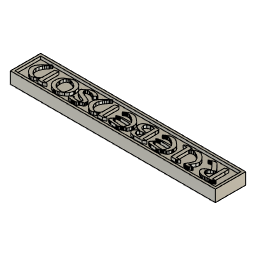
RuebensonBrandingIron v5 (Autodesk Fusion 360 design; units mm, degrees)
Autodesk Fusion 360 part; units mm, degrees
(part 1 of 2)
sketch "Sketch1" plane through (0, 0, 0) normal (0, 0, 1) x (1, 0, 0)
  line L0 (0, 0) -> (223.52, 0)
  line L1 (223.52, 0) -> (223.52, 33.02)
  line L2 (223.52, 33.02) -> (0, 33.02)
  line L3 (0, 33.02) -> (0, 0)
  dimension "d1" = 223.52
  dimension "d2" = 33.02
  constraint horizontal L0
  constraint vertical L1
  constraint horizontal L2
  constraint vertical L3
  constraint coincident L0.start L3.end
  measures "d1" distance of L0.start L0.end
  measures "d2" distance of L0.start L2.end
extrude "Extrude1" add sketch "Sketch1" along normal blind 12.7
sketch "Sketch4" plane through (0, 0, 12.7) normal (0, 0, 1) x (-1, 0, 0)
  line L0 (0, -33.02) -> (0, 0)
  line L1 (0, 0) -> (-223.52, 0)
  line L2 (-223.52, 0) -> (-223.52, -33.02)
  line L3 (-223.52, -33.02) -> (0, -33.02)
  spline S0 degree 3 poles (-115.0505, -8.6824) (-114.8396, -8.6121) (-114.6287, -8.533) (-114.4177, -8.4451) knots 0 0 0 0 1 1 1 1
  spline S1 degree 3 poles (-110.8582, -6.4148) (-110.7879, -6.3973) (-110.7132, -6.3885) (-110.6341, -6.3885) knots 0 0 0 0 1 1 1 1
  spline S2 degree 3 poles (-114.4177, -8.4451) (-114.2068, -8.3572) (-114.0047, -8.2693) (-113.8113, -8.1814) knots 0 0 0 0 1 1 1 1
  line L4 (-132.9807, -8.1814) -> (-132.9807, -14.2985)
  spline S3 degree 3 poles (-109.6322, -6.4148) (-109.3597, -6.4324) (-109.0741, -6.4588) (-108.7753, -6.4939) knots 0 0 0 0 1 1 1 1
  spline S4 degree 3 poles (-131.3855, -15.8805) (-131.5525, -15.8629) (-131.7239, -15.8541) (-131.8997, -15.8541) knots 0 0 0 0 1 1 1 1
  spline S5 degree 3 poles (-130.0276, -14.3249) (-129.0784, -14.2546) (-128.1952, -14.0173) (-127.3778, -13.613) knots 0 0 0 0 1 1 1 1
  line L5 (-132.9807, -23.395) -> (-132.9807, -23.4082)
  spline S6 degree 3 poles (-130.7923, -14.3249) (-130.6692, -14.3424) (-130.5418, -14.3468) (-130.41, -14.3381) knots 0 0 0 0 1 1 1 1
  line L6 (-136.4084, -24.7661) -> (-136.4084, -24.7397)
  line L7 (-132.9807, -15.775) -> (-132.9807, -23.3159)
  spline S7 degree 3 poles (-116.6325, -9.2229) (-116.1404, -9.0735) (-115.613, -8.8933) (-115.0505, -8.6824) knots 0 0 0 0 1 1 1 1
  line L8 (-131.0032, -8.2078) -> (-132.9807, -8.1814)
  arc A0 (-108.7753, -6.4939) -> (-108.5643, -6.5335) centre (-108.3426, -4.7686) ccw
  line L9 (-132.9807, -23.3555) -> (-132.9807, -23.395)
  line L10 (-131.8997, -15.8278) -> (-132.9807, -15.775)
  spline S8 degree 3 poles (-133.719, -25.9262) (-134.967, -25.9438) (-135.7273, -25.9131) (-135.9997, -25.834) knots 0 0 0 0 1 1 1 1
  line L11 (-131.8997, -15.8541) -> (-131.8997, -15.8278)
  spline S9 degree 3 poles (-113.8113, -8.1814) (-113.6179, -8.0759) (-113.4246, -7.9617) (-113.2312, -7.8386) knots 0 0 0 0 1 1 1 1
  spline S10 degree 3 poles (-132.9807, -23.5664) (-132.9807, -23.6279) (-132.9719, -23.6851) (-132.9544, -23.7378) knots 0 0 0 0 1 1 1 1
  arc A1 (-131.3855, -15.8805) -> (-130.8714, -15.9332) centre (-120.9987, 82.8585) ccw
  spline S11 degree 3 poles (-113.2312, -7.8386) (-113.0379, -7.7156) (-112.8533, -7.5926) (-112.6775, -7.4695) knots 0 0 0 0 1 1 1 1
  line L12 (-125.9935, -11.5827) -> (-125.9935, -11.5168)
  spline S12 degree 3 poles (-110.3836, -6.3885) (-110.1551, -6.3885) (-109.9046, -6.3973) (-109.6322, -6.4148) knots 0 0 0 0 1 1 1 1
  spline S13 degree 3 poles (-125.9672, -11.3191) (-125.9672, -10.4226) (-126.3715, -9.7283) (-127.18, -9.2361) knots 0 0 0 0 1 1 1 1
  line L13 (-117.4499, -9.4998) -> (-117.5026, -9.5261)
  line L14 (-132.9807, -23.4082) -> (-132.9807, -23.4214)
  line L15 (-133.1653, -25.9262) -> (-133.4553, -25.9262)
  spline S14 degree 3 poles (-125.9935, -11.5168) (-125.9935, -11.4904) (-125.9847, -11.4685) (-125.9672, -11.4509) knots 0 0 0 0 1 1 1 1
  line L16 (-132.9807, -14.2985) -> (-130.7923, -14.3249)
  line L17 (-110.6341, -6.3885) -> (-110.3836, -6.3885)
  spline S15 degree 3 poles (-130.41, -14.3381) (-130.2781, -14.3293) (-130.1507, -14.3249) (-130.0276, -14.3249) knots 0 0 0 0 1 1 1 1
  spline S16 degree 3 poles (-127.3778, -13.613) (-126.5604, -13.2087) (-126.099, -12.5319) (-125.9935, -11.5827) knots 0 0 0 0 1 1 1 1
  spline S17 degree 3 poles (-117.5026, -9.5261) (-117.4148, -9.4734) (-117.1247, -9.3723) (-116.6325, -9.2229) knots 0 0 0 0 1 1 1 1
  line L18 (-132.9807, -23.4214) -> (-132.9807, -23.5664)
  line L19 (-132.9807, -23.3159) -> (-132.9807, -23.3555)
  spline S18 degree 3 poles (-111.6888, -6.7708) (-111.3812, -6.5511) (-111.1043, -6.4324) (-110.8582, -6.4148) knots 0 0 0 0 1 1 1 1
  spline S19 degree 3 poles (-112.6775, -7.4695) (-112.326, -7.2234) (-111.9964, -6.9905) (-111.6888, -6.7708) knots 0 0 0 0 1 1 1 1
  arc A2 (-132.9544, -23.7378) -> (-132.9016, -23.9355) centre (-126.9769, -22.2497) ccw
  line L20 (-124.2533, -20.9166) -> (-124.2533, -20.8243)
  spline S20 degree 3 poles (-123.6601, -23.54) (-125.62, -24.6387) (-127.7777, -25.3637) (-130.1331, -25.7153) knots 0 0 0 0 1 1 1 1
  line L21 (-131.7151, -24.3179) -> (-128.7884, -24.2915)
  spline S21 degree 3 poles (-124.2533, -20.7584) (-124.3588, -19.0885) (-125.0883, -17.902) (-126.4418, -17.1988) knots 0 0 0 0 1 1 1 1
  line L22 (-124.2533, -20.8243) -> (-124.2533, -20.7584)
  line L23 (-137.2785, -6.2303) -> (-128.4456, -6.0984)
  spline S22 degree 3 poles (-131.6624, -25.8735) (-132.1721, -25.9087) (-132.6731, -25.9262) (-133.1653, -25.9262) knots 0 0 0 0 1 1 1 1
  spline S23 degree 3 poles (-126.4418, -17.1988) (-127.7953, -16.4957) (-129.2718, -16.0739) (-130.8714, -15.9332) knots 0 0 0 0 1 1 1 1
  line L24 (-133.4553, -25.9262) -> (-133.719, -25.9262)
  spline S24 degree 3 poles (-125.5453, -23.2368) (-124.684, -22.604) (-124.2533, -21.8306) (-124.2533, -20.9166) knots 0 0 0 0 1 1 1 1
  line L25 (-131.847, -24.3179) -> (-131.781, -24.3179)
  spline S25 degree 3 poles (-128.7884, -24.2915) (-128.7181, -24.3091) (-128.6478, -24.3179) (-128.5775, -24.3179) knots 0 0 0 0 1 1 1 1
  spline S26 degree 3 poles (-132.9016, -23.9355) (-132.884, -23.9971) (-132.8577, -24.0454) (-132.8225, -24.0806) knots 0 0 0 0 1 1 1 1
  spline S27 degree 3 poles (-132.4138, -24.2915) (-132.2468, -24.3091) (-132.0667, -24.3179) (-131.8733, -24.3179) knots 0 0 0 0 1 1 1 1
  line L26 (-131.781, -24.3179) -> (-131.7151, -24.3179)
  spline S28 degree 3 poles (-132.8225, -24.0806) (-132.7171, -24.2036) (-132.5808, -24.2739) (-132.4138, -24.2915) knots 0 0 0 0 1 1 1 1
  spline S29 degree 3 poles (-128.3665, -24.2915) (-127.347, -24.2212) (-126.4066, -23.8696) (-125.5453, -23.2368) knots 0 0 0 0 1 1 1 1
  arc A3 (-131.6624, -25.8735) -> (-130.1331, -25.7153) centre (-133.2155, -3.3893) ccw
  spline S30 degree 3 poles (-135.9997, -25.834) (-136.2722, -25.7549) (-136.4084, -25.3989) (-136.4084, -24.7661) knots 0 0 0 0 1 1 1 1
  spline S31 degree 3 poles (-127.9579, -6.138) (-127.7909, -6.1468) (-127.6283, -6.16) (-127.4701, -6.1775) knots 0 0 0 0 1 1 1 1
  spline S32 degree 3 poles (-128.5775, -24.3179) (-128.5072, -24.3179) (-128.4369, -24.3091) (-128.3665, -24.2915) knots 0 0 0 0 1 1 1 1
  line L27 (-131.8733, -24.3179) -> (-131.847, -24.3179)
  spline S33 degree 3 poles (-127.4701, -6.1775) (-126.2748, -6.283) (-125.1674, -6.6346) (-124.1479, -7.2322) knots 0 0 0 0 1 1 1 1
  line L28 (-136.4348, -21.6021) -> (-136.5402, -8.1023)
  spline S34 degree 3 poles (-161.1168, -9.5657) (-161.0992, -9.5569) (-161.0817, -9.5437) (-161.0641, -9.5261) knots 0 0 0 0 1 1 1 1
  line L29 (-140.7325, -8.1814) -> (-137.2785, -6.2303)
  arc A4 (-115.5251, -12.6901) -> (-115.6042, -13.3229) centre (-107.8557, -13.9702) ccw
  spline S35 degree 3 poles (-114.9055, -10.1853) (-115.1956, -10.9587) (-115.4021, -11.7937) (-115.5251, -12.6901) knots 0 0 0 0 1 1 1 1
  spline S36 degree 3 poles (-109.2103, -22.1953) (-108.8324, -22.4151) (-108.4501, -22.6128) (-108.0633, -22.7886) knots 0 0 0 0 1 1 1 1
  spline S37 degree 3 poles (-110.3836, -21.4966) (-109.9793, -21.7427) (-109.5882, -21.9756) (-109.2103, -22.1953) knots 0 0 0 0 1 1 1 1
  spline S38 degree 3 poles (-115.6042, -13.3229) (-115.6218, -13.5339) (-115.6306, -13.736) (-115.6306, -13.9294) knots 0 0 0 0 1 1 1 1
  spline S39 degree 3 poles (-112.8357, -19.5455) (-112.4666, -19.897) (-112.0755, -20.2398) (-111.6624, -20.5738) knots 0 0 0 0 1 1 1 1
  spline S40 degree 3 poles (-111.6624, -20.5738) (-111.2493, -20.9078) (-110.8231, -21.2154) (-110.3836, -21.4966) knots 0 0 0 0 1 1 1 1
  spline S41 degree 3 poles (-114.8923, -17.1197) (-114.699, -17.4361) (-114.4221, -17.8053) (-114.0618, -18.2271) knots 0 0 0 0 1 1 1 1
  line L30 (-136.4084, -24.7397) -> (-136.4348, -21.6021)
  line L31 (-161.0641, -9.5261) -> (-161.0641, -9.4998)
  line L32 (-136.5402, -8.1023) -> (-140.7325, -8.1814)
  spline S42 degree 3 poles (-161.1696, -9.6052) (-161.152, -9.5876) (-161.1344, -9.5745) (-161.1168, -9.5657) knots 0 0 0 0 1 1 1 1
  arc A5 (-162.7252, -14.7467) -> (-162.7516, -15.1686) centre (-159.3535, -15.1692) ccw
  spline S43 degree 3 poles (-113.9168, -8.7878) (-114.2859, -8.946) (-114.6155, -9.4119) (-114.9055, -10.1853) knots 0 0 0 0 1 1 1 1
  spline S44 degree 3 poles (-162.6593, -14.0876) (-162.6329, -13.8591) (-162.5934, -13.6393) (-162.5406, -13.4284) knots 0 0 0 0 1 1 1 1
  spline S45 degree 3 poles (-162.5406, -13.4284) (-162.4, -12.6022) (-162.2023, -11.8288) (-161.9474, -11.1081) knots 0 0 0 0 1 1 1 1
  spline S46 degree 3 poles (-128.4456, -6.0984) (-128.2874, -6.116) (-128.1248, -6.1292) (-127.9579, -6.138) knots 0 0 0 0 1 1 1 1
  spline S47 degree 3 poles (-161.9474, -11.1081) (-161.6925, -10.3874) (-161.4332, -9.8865) (-161.1696, -9.6052) knots 0 0 0 0 1 1 1 1
  spline S48 degree 3 poles (-162.7252, -14.7467) (-162.7076, -14.5358) (-162.6856, -14.3161) (-162.6593, -14.0876) knots 0 0 0 0 1 1 1 1
  line L33 (-198.044, -26.0053) -> (-198.1231, -26.0053)
  spline S49 degree 3 poles (-9.0744, -10.9763) (-8.0549, -12.3649) (-7.5452, -13.8327) (-7.5452, -15.3795) knots 0 0 0 0 1 1 1 1
  spline S50 degree 3 poles (-203.1987, -21.9976) (-203.4184, -21.7691) (-203.6601, -21.5142) (-203.9237, -21.233) knots 0 0 0 0 1 1 1 1
  spline S51 degree 3 poles (-201.9199, -23.3159) (-202.1308, -23.105) (-202.3329, -22.8941) (-202.5263, -22.6831) knots 0 0 0 0 1 1 1 1
  spline S52 degree 3 poles (-202.4077, -16.9484) (-202.2055, -17.2032) (-202.0078, -17.4449) (-201.8144, -17.6734) knots 0 0 0 0 1 1 1 1
  spline S53 degree 3 poles (-8.2571, -18.3985) (-8.7317, -19.3741) (-9.259, -20.2486) (-9.8391, -21.022) knots 0 0 0 0 1 1 1 1
  spline S54 degree 3 poles (-202.5527, -22.6568) (-202.7636, -22.4458) (-202.9789, -22.2261) (-203.1987, -21.9976) knots 0 0 0 0 1 1 1 1
  spline S55 degree 3 poles (-204.1083, -5.8875) (-203.7216, -5.8875) (-203.2514, -5.9315) (-202.6977, -6.0193) knots 0 0 0 0 1 1 1 1
  spline S56 degree 3 poles (-22.0469, -9.1834) (-22.6797, -9.8162) (-23.1103, -10.5017) (-23.3388, -11.24) knots 0 0 0 0 1 1 1 1
  spline S57 degree 3 poles (-14.4928, -6.4017) (-13.8336, -6.6917) (-13.1525, -7.0828) (-12.4494, -7.575) knots 0 0 0 0 1 1 1 1
  line L34 (-194.8008, -24.0015) -> (-194.7481, -24.0015)
  spline S58 degree 3 poles (-196.9893, -10.449) (-196.9717, -10.5193) (-196.9629, -10.5896) (-196.9629, -10.6599) knots 0 0 0 0 1 1 1 1
  line L35 (-223.52, 0) -> (-223.52, -33.02)
  spline S59 degree 3 poles (-202.6977, -6.0193) (-202.144, -6.1072) (-201.5771, -6.2479) (-200.997, -6.4412) knots 0 0 0 0 1 1 1 1
  spline S60 degree 3 poles (-200.997, -6.4412) (-200.0654, -6.74) (-199.1997, -7.2102) (-198.3999, -7.8518) knots 0 0 0 0 1 1 1 1
  spline S61 degree 3 poles (-200.9707, -24.3706) (-201.0234, -24.3003) (-201.0717, -24.2388) (-201.1157, -24.186) knots 0 0 0 0 1 1 1 1
  line L36 (-194.9063, -24.0015) -> (-194.8536, -24.0015)
  spline S62 degree 3 poles (-205.453, -19.4664) (-205.4706, -19.4488) (-205.4926, -19.4224) (-205.5189, -19.3873) knots 0 0 0 0 1 1 1 1
  spline S63 degree 3 poles (-198.4263, -13.5866) (-199.4018, -14.2897) (-200.4697, -14.9137) (-201.6298, -15.4586) knots 0 0 0 0 1 1 1 1
  line L37 (-202.5263, -22.6831) -> (-202.5395, -22.6831)
  spline S64 degree 3 poles (-203.0536, -16.0914) (-202.8251, -16.4078) (-202.6098, -16.6935) (-202.4077, -16.9484) knots 0 0 0 0 1 1 1 1
  arc A6 (-201.6694, -17.8448) -> (-201.5244, -18.0162) centre (-200.5632, -17.0559) ccw
  arc A7 (-202.1176, -15.6959) -> (-202.6054, -15.9069) centre (-191.6517, -40.5679) ccw
  spline S65 degree 3 poles (-16.1935, -5.9666) (-15.7189, -5.9666) (-15.152, -6.1116) (-14.4928, -6.4017) knots 0 0 0 0 1 1 1 1
  arc A8 (-205.453, -19.4664) -> (-204.517, -20.5474) centre (191.9498, 323.6805) ccw
  spline S66 degree 3 poles (-193.7594, -23.8564) (-193.5045, -23.7773) (-193.2716, -23.6939) (-193.0606, -23.606) knots 0 0 0 0 1 1 1 1
  line L38 (-202.6054, -15.9069) -> (-203.0536, -16.0914)
  line L39 (-223.52, -33.02) -> (0, -33.02)
  arc A9 (-202.1176, -15.6959) -> (-201.6298, -15.4586) centre (-204.0555, -11.0925) ccw
  spline S67 degree 3 poles (-196.9629, -10.8708) (-196.9629, -11.9782) (-197.4507, -12.8835) (-198.4263, -13.5866) knots 0 0 0 0 1 1 1 1
  spline S68 degree 3 poles (-198.3999, -7.8518) (-197.6001, -8.4934) (-197.1299, -9.3591) (-196.9893, -10.449) knots 0 0 0 0 1 1 1 1
  spline S69 degree 3 poles (-194.5372, -24.0015) (-194.2735, -23.9839) (-194.0142, -23.9355) (-193.7594, -23.8564) knots 0 0 0 0 1 1 1 1
  arc A10 (-19.753, -7.9573) -> (-20.0166, -7.9968) centre (-19.4806, -10.6714) ccw
  line L40 (0, -33.02) -> (0, 0)
  spline S70 degree 3 poles (-20.0166, -7.9968) (-20.7373, -8.155) (-21.4141, -8.5505) (-22.0469, -9.1834) knots 0 0 0 0 1 1 1 1
  arc A11 (-19.4893, -7.9441) -> (-19.753, -7.9573) centre (-19.4891, -10.5923) ccw
  line L41 (-194.6426, -24.0015) -> (-194.5372, -24.0015)
  spline S71 degree 3 poles (-202.5395, -22.6831) (-202.5483, -22.6831) (-202.5527, -22.6743) (-202.5527, -22.6568) knots 0 0 0 0 1 1 1 1
  spline S72 degree 3 poles (-201.2607, -24.0278) (-201.4892, -23.7642) (-201.7089, -23.5269) (-201.9199, -23.3159) knots 0 0 0 0 1 1 1 1
  spline S73 degree 3 poles (-7.5452, -15.3795) (-7.5452, -16.4166) (-7.7825, -17.423) (-8.2571, -18.3985) knots 0 0 0 0 1 1 1 1
  line L42 (-197.9649, -26.0053) -> (-198.044, -26.0053)
  line L43 (-197.8989, -26.0053) -> (-197.9649, -26.0053)
  line L44 (-196.9629, -10.6599) -> (-196.9629, -10.8708)
  spline S74 degree 3 poles (-9.8391, -21.022) (-10.2258, -21.5318) (-10.5949, -21.9756) (-10.9465, -22.3535) knots 0 0 0 0 1 1 1 1
  line L45 (0, 0) -> (-223.52, 0)
  spline S75 degree 3 poles (-12.4494, -7.575) (-11.2189, -8.4539) (-10.0939, -9.5876) (-9.0744, -10.9763) knots 0 0 0 0 1 1 1 1
  arc A12 (-201.6694, -17.8448) -> (-201.8144, -17.6734) centre (-202.7756, -18.6338) ccw
  spline S76 degree 3 poles (-199.7182, -25.4516) (-200.1841, -25.1177) (-200.6015, -24.7573) (-200.9707, -24.3706) knots 0 0 0 0 1 1 1 1
  spline S77 degree 3 poles (-198.1231, -26.0053) (-198.7207, -25.9702) (-199.2524, -25.7856) (-199.7182, -25.4516) knots 0 0 0 0 1 1 1 1
  spline S78 degree 3 poles (-201.1157, -24.186) (-201.1596, -24.1333) (-201.208, -24.0806) (-201.2607, -24.0278) knots 0 0 0 0 1 1 1 1
  line L46 (-194.7481, -24.0015) -> (-194.6426, -24.0015)
  spline S79 degree 3 poles (-203.9237, -21.233) (-204.0292, -21.1099) (-204.227, -20.8814) (-204.517, -20.5474) knots 0 0 0 0 1 1 1 1
  line L47 (-194.959, -24.0015) -> (-194.9063, -24.0015)
  spline S80 degree 3 poles (-195.9082, -23.7642) (-195.6446, -23.9048) (-195.3282, -23.9839) (-194.959, -24.0015) knots 0 0 0 0 1 1 1 1
  line L48 (-194.8536, -24.0015) -> (-194.8008, -24.0015)
  spline S81 degree 3 poles (-23.3388, -11.24) (-23.374, -11.3982) (-23.4048, -11.552) (-23.4311, -11.7014) knots 0 0 0 0 1 1 1 1
  line L49 (-204.1479, -5.8875) -> (-204.1083, -5.8875)
  spline S82 degree 3 poles (-196.9102, -22.9204) (-196.875, -22.9907) (-196.8355, -23.0435) (-196.7915, -23.0786) knots 0 0 0 0 1 1 1 1
  spline S83 degree 3 poles (-196.7915, -23.0786) (-196.7476, -23.1138) (-196.708, -23.1577) (-196.6729, -23.2105) knots 0 0 0 0 1 1 1 1
  arc A13 (-199.4414, -20.3497) -> (-198.8086, -20.9957) centre (-167.4667, 10.3396) ccw
  spline S84 degree 3 poles (-67.3132, -8.3923) (-67.1902, -8.3045) (-67.0628, -8.2078) (-66.9309, -8.1023) knots 0 0 0 0 1 1 1 1
  spline S85 degree 3 poles (-196.6729, -23.2105) (-196.4268, -23.439) (-196.1719, -23.6235) (-195.9082, -23.7642) knots 0 0 0 0 1 1 1 1
  spline S86 degree 3 poles (-70.4772, -10.1062) (-70.4245, -10.071) (-70.363, -10.0271) (-70.2927, -9.9744) knots 0 0 0 0 1 1 1 1
  spline S87 degree 3 poles (-200.8652, -18.7677) (-200.6367, -19.0225) (-200.3906, -19.2994) (-200.1269, -19.5982) knots 0 0 0 0 1 1 1 1
  arc A14 (-66.9309, -8.1023) -> (-66.5486, -7.7859) centre (-76.0785, 3.3402) ccw
  line L50 (-88.8919, -12.1364) -> (-88.8919, -24.6079)
  spline S88 degree 3 poles (-68.6052, -15.4455) (-68.6228, -15.4367) (-68.6404, -15.4235) (-68.6579, -15.4059) knots 0 0 0 0 1 1 1 1
  spline S89 degree 3 poles (-68.6579, -15.4059) (-69.0974, -15.2301) (-69.5061, -15.028) (-69.884, -14.7995) knots 0 0 0 0 1 1 1 1
  spline S90 degree 3 poles (-59.2714, -20.8375) (-59.3417, -20.5738) (-59.4296, -20.3145) (-59.535, -20.0596) knots 0 0 0 0 1 1 1 1
  line L51 (-198.769, -21.0088) -> (-198.7559, -21.022)
  spline S91 degree 3 poles (-70.1081, -24.8716) (-70.4948, -24.6958) (-70.8156, -24.5156) (-71.0705, -24.3311) knots 0 0 0 0 1 1 1 1
  spline S92 degree 3 poles (-70.2927, -9.9744) (-70.0114, -9.8337) (-69.6071, -9.658) (-69.0798, -9.447) knots 0 0 0 0 1 1 1 1
  spline S93 degree 3 poles (-60.6424, -18.8336) (-60.9413, -18.6226) (-61.5916, -18.315) (-62.5936, -17.9107) knots 0 0 0 0 1 1 1 1
  spline S94 degree 3 poles (-65.6389, -26.1372) (-65.9466, -26.102) (-66.2498, -26.0581) (-66.5486, -26.0053) knots 0 0 0 0 1 1 1 1
  spline S95 degree 3 poles (-69.0007, -20.9693) (-68.9831, -20.9341) (-68.9612, -20.9034) (-68.9348, -20.877) knots 0 0 0 0 1 1 1 1
  spline S96 degree 3 poles (-68.5525, -15.4323) (-68.57, -15.4498) (-68.5876, -15.4542) (-68.6052, -15.4455) knots 0 0 0 0 1 1 1 1
  spline S97 degree 3 poles (-64.7293, -26.1899) (-65.0281, -26.1899) (-65.3313, -26.1723) (-65.6389, -26.1372) knots 0 0 0 0 1 1 1 1
  line L52 (-197.3584, -22.4722) -> (-196.9102, -22.9204)
  spline S98 degree 3 poles (-58.5067, -10.0271) (-58.5946, -9.8162) (-58.9154, -9.6316) (-59.4691, -9.4734) knots 0 0 0 0 1 1 1 1
  spline S99 degree 3 poles (-66.5486, -26.0053) (-67.2166, -25.8999) (-67.8581, -25.7417) (-68.4734, -25.5307) knots 0 0 0 0 1 1 1 1
  spline S100 degree 3 poles (-200.1269, -19.5982) (-199.8808, -19.8795) (-199.6523, -20.1299) (-199.4414, -20.3497) knots 0 0 0 0 1 1 1 1
  spline S101 degree 3 poles (-65.3885, -6.8499) (-65.0193, -6.5599) (-64.6766, -6.3709) (-64.3602, -6.283) knots 0 0 0 0 1 1 1 1
  spline S102 degree 3 poles (-70.8596, -13.2702) (-70.9035, -12.9714) (-70.9343, -12.6638) (-70.9518, -12.3474) knots 0 0 0 0 1 1 1 1
  spline S103 degree 3 poles (-64.1624, -6.2698) (-64.0306, -6.261) (-63.8504, -6.2479) (-63.6219, -6.2303) knots 0 0 0 0 1 1 1 1
  spline S104 degree 3 poles (-68.4734, -25.5307) (-69.0886, -25.3198) (-69.6335, -25.1001) (-70.1081, -24.8716) knots 0 0 0 0 1 1 1 1
  spline S105 degree 3 poles (-59.4691, -9.4734) (-60.0228, -9.3152) (-60.6337, -9.1746) (-61.3016, -9.0515) knots 0 0 0 0 1 1 1 1
  line L53 (-64.5975, -26.1899) -> (-64.6238, -26.1899)
  line L54 (-64.3865, -26.1899) -> (-64.5447, -26.1899)
  line L55 (-64.3602, -6.283) -> (-64.1624, -6.2698)
  spline S106 degree 3 poles (-68.8689, -20.8111) (-68.781, -20.7408) (-68.7019, -20.688) (-68.6316, -20.6529) knots 0 0 0 0 1 1 1 1
  spline S107 degree 3 poles (-66.5486, -7.7859) (-66.1443, -7.4519) (-65.7576, -7.1399) (-65.3885, -6.8499) knots 0 0 0 0 1 1 1 1
  spline S108 degree 3 poles (-68.6316, -20.6529) (-68.5613, -20.6177) (-68.4997, -20.6441) (-68.447, -20.732) knots 0 0 0 0 1 1 1 1
  spline S109 degree 3 poles (-58.4936, -10.0666) (-58.5023, -10.0578) (-58.5067, -10.0447) (-58.5067, -10.0271) knots 0 0 0 0 1 1 1 1
  spline S110 degree 3 poles (-59.535, -20.0596) (-59.6405, -19.8048) (-59.7811, -19.5894) (-59.9569, -19.4137) knots 0 0 0 0 1 1 1 1
  spline S111 degree 3 poles (-198.0967, -21.7076) (-197.8682, -21.9361) (-197.6221, -22.1909) (-197.3584, -22.4722) knots 0 0 0 0 1 1 1 1
  spline S112 degree 3 poles (-68.447, -20.732) (-68.4294, -20.7496) (-68.4206, -20.7715) (-68.4206, -20.7979) knots 0 0 0 0 1 1 1 1
  spline S113 degree 3 poles (-63.4901, -26.1504) (-63.7186, -26.1591) (-63.9647, -26.1723) (-64.2283, -26.1899) knots 0 0 0 0 1 1 1 1
  spline S114 degree 3 poles (-70.6618, -14.0348) (-70.7497, -13.8239) (-70.8156, -13.569) (-70.8596, -13.2702) knots 0 0 0 0 1 1 1 1
  spline S115 degree 3 poles (-71.0705, -24.3311) (-71.3254, -24.1465) (-71.4704, -23.9927) (-71.5055, -23.8696) knots 0 0 0 0 1 1 1 1
  spline S116 degree 3 poles (-59.1659, -21.4834) (-59.1835, -21.2813) (-59.2186, -21.066) (-59.2714, -20.8375) knots 0 0 0 0 1 1 1 1
  spline S117 degree 3 poles (-70.6091, -10.2117) (-70.5739, -10.1765) (-70.53, -10.1413) (-70.4772, -10.1062) knots 0 0 0 0 1 1 1 1
  spline S118 degree 3 poles (-198.7559, -21.022) (-198.5449, -21.2505) (-198.3252, -21.479) (-198.0967, -21.7076) knots 0 0 0 0 1 1 1 1
  line L56 (-88.8919, -24.6079) -> (-92.4251, -25.9262)
  spline S119 degree 3 poles (-59.9569, -19.4137) (-60.1151, -19.2379) (-60.3436, -19.0445) (-60.6424, -18.8336) knots 0 0 0 0 1 1 1 1
  line L57 (-71.5055, -23.8301) -> (-71.5055, -23.8169)
  spline S120 degree 3 poles (-69.884, -14.7995) (-70.2619, -14.571) (-70.5212, -14.3161) (-70.6618, -14.0348) knots 0 0 0 0 1 1 1 1
  line L58 (-64.6766, -26.1899) -> (-64.7293, -26.1899)
  spline S121 degree 3 poles (-88.8524, -11.7014) (-88.8788, -11.8508) (-88.8919, -11.9958) (-88.8919, -12.1364) knots 0 0 0 0 1 1 1 1
  spline S122 degree 3 poles (-59.1395, -22.0503) (-59.1395, -21.8745) (-59.1483, -21.6856) (-59.1659, -21.4834) knots 0 0 0 0 1 1 1 1
  line L59 (-70.7145, -10.2117) -> (-70.6091, -10.2117)
  spline S123 degree 3 poles (-198.8086, -20.9957) (-198.791, -20.9957) (-198.7778, -21.0001) (-198.769, -21.0088) knots 0 0 0 0 1 1 1 1
  spline S124 degree 3 poles (-69.0798, -9.447) (-68.5525, -9.2361) (-67.9636, -8.8845) (-67.3132, -8.3923) knots 0 0 0 0 1 1 1 1
  line L60 (-64.6238, -26.1899) -> (-64.6766, -26.1899)
  line L61 (-64.2283, -26.1899) -> (-64.3865, -26.1899)
  line L62 (-62.5936, -17.9107) -> (-68.5525, -15.4323)
  line L63 (-64.5447, -26.1899) -> (-64.5975, -26.1899)
  line L64 (-71.5055, -23.8696) -> (-71.5055, -23.8301)
  arc A15 (-63.4901, -26.1504) -> (-62.8045, -26.0844) centre (-63.7234, -20.1261) ccw
  line L65 (-68.9348, -20.877) -> (-68.8689, -20.8111)
  spline S125 degree 3 poles (-69.093, -21.0748) (-69.0666, -21.0396) (-69.0359, -21.0044) (-69.0007, -20.9693) knots 0 0 0 0 1 1 1 1
  spline S126 degree 3 poles (-69.1853, -21.1539) (-69.1501, -21.1363) (-69.1194, -21.1099) (-69.093, -21.0748) knots 0 0 0 0 1 1 1 1
  line L66 (-71.0441, -23.0654) -> (-70.9518, -22.9732)
  line L67 (-71.1364, -23.1577) -> (-71.0441, -23.0654)
  line L68 (-70.9518, -22.9732) -> (-69.1853, -21.1539)
  spline S127 degree 3 poles (-71.4396, -23.4741) (-71.3781, -23.3862) (-71.3034, -23.3071) (-71.2155, -23.2368) knots 0 0 0 0 1 1 1 1
  spline S128 degree 3 poles (-55.7382, -19.8619) (-55.7207, -19.897) (-55.7119, -19.9366) (-55.7119, -19.9805) knots 0 0 0 0 1 1 1 1
  spline S129 degree 3 poles (-56.8456, -17.1988) (-56.5644, -17.5504) (-56.3183, -17.9591) (-56.1074, -18.4249) knots 0 0 0 0 1 1 1 1
  spline S130 degree 3 poles (-58.744, -15.6432) (-57.9179, -16.1002) (-57.2851, -16.6188) (-56.8456, -17.1988) knots 0 0 0 0 1 1 1 1
  line L69 (-67.5769, -11.2927) -> (-67.5769, -11.3454)
  spline S131 degree 3 poles (-61.4334, -14.3776) (-60.4667, -14.7643) (-59.5702, -15.1862) (-58.744, -15.6432) knots 0 0 0 0 1 1 1 1
  line L70 (-65.4412, -12.8483) -> (-61.4334, -14.3776)
  spline S132 degree 3 poles (-67.0496, -12.0441) (-66.7507, -12.2639) (-66.2146, -12.5319) (-65.4412, -12.8483) knots 0 0 0 0 1 1 1 1
  spline S133 degree 3 poles (-71.176, -23.1841) (-71.1672, -23.1665) (-71.154, -23.1577) (-71.1364, -23.1577) knots 0 0 0 0 1 1 1 1
  line L71 (-71.5319, -23.7773) -> (-71.5319, -23.7642)
  spline S134 degree 3 poles (-71.5055, -23.8169) (-71.5231, -23.7993) (-71.5319, -23.7861) (-71.5319, -23.7773) knots 0 0 0 0 1 1 1 1
  spline S135 degree 3 poles (-56.1074, -18.4249) (-55.8964, -18.8907) (-55.7734, -19.3697) (-55.7382, -19.8619) knots 0 0 0 0 1 1 1 1
  spline S136 degree 3 poles (-71.2155, -23.2368) (-71.1979, -23.2193) (-71.1848, -23.2017) (-71.176, -23.1841) knots 0 0 0 0 1 1 1 1
  spline S137 degree 3 poles (-71.5319, -23.7642) (-71.5319, -23.6587) (-71.5012, -23.562) (-71.4396, -23.4741) knots 0 0 0 0 1 1 1 1
  line L72 (-55.7119, -19.9805) -> (-55.7119, -20.0992)
  spline S138 degree 3 poles (-58.5199, -10.3171) (-58.4936, -10.2644) (-58.4804, -10.2117) (-58.4804, -10.1589) knots 0 0 0 0 1 1 1 1
  spline S139 degree 3 poles (-67.5769, -11.4245) (-67.5242, -11.6179) (-67.3484, -11.8244) (-67.0496, -12.0441) knots 0 0 0 0 1 1 1 1
  line L73 (-67.5769, -11.2136) -> (-67.5769, -11.2927)
  line L74 (-67.5769, -11.0818) -> (-67.5769, -11.2136)
  spline S140 degree 3 poles (-60.7215, -25.0561) (-61.0731, -25.4077) (-61.3543, -25.6274) (-61.5653, -25.7153) knots 0 0 0 0 1 1 1 1
  line L75 (-67.6033, -10.7654) -> (-67.6033, -10.9367)
  arc A16 (-59.1264, -23.5269) -> (-59.5614, -23.9487) centre (-45.4173, -38.0996) ccw
  spline S141 degree 3 poles (-56.3974, -21.4571) (-56.749, -21.712) (-57.1445, -21.9888) (-57.5839, -22.2876) knots 0 0 0 0 1 1 1 1
  spline S142 degree 3 poles (-55.7514, -20.5342) (-55.7778, -20.6836) (-55.8085, -20.8287) (-55.8437, -20.9693) knots 0 0 0 0 1 1 1 1
  line L76 (-58.4804, -10.1589) -> (-58.4804, -10.1194)
  line L77 (-58.4804, -10.1194) -> (-58.4804, -10.0798)
  spline S143 degree 3 poles (-61.5653, -25.7153) (-61.7938, -25.8208) (-62.0091, -25.8999) (-62.2113, -25.9526) knots 0 0 0 0 1 1 1 1
  spline S144 degree 3 poles (-55.8437, -20.9693) (-55.8613, -21.0396) (-56.0458, -21.2022) (-56.3974, -21.4571) knots 0 0 0 0 1 1 1 1
  spline S145 degree 3 poles (-58.6781, -10.6467) (-58.6518, -10.5852) (-58.6298, -10.5281) (-58.6122, -10.4753) knots 0 0 0 0 1 1 1 1
  spline S146 degree 3 poles (-62.2113, -25.9526) (-62.4134, -26.0053) (-62.6112, -26.0493) (-62.8045, -26.0844) knots 0 0 0 0 1 1 1 1
  spline S147 degree 3 poles (-58.5858, -10.4753) (-58.5683, -10.4226) (-58.5463, -10.3699) (-58.5199, -10.3171) knots 0 0 0 0 1 1 1 1
  line L78 (-58.6122, -10.4753) -> (-58.5858, -10.4753)
  spline S148 degree 3 poles (-58.7177, -10.8181) (-58.7177, -10.7654) (-58.7045, -10.7082) (-58.6781, -10.6467) knots 0 0 0 0 1 1 1 1
  spline S149 degree 3 poles (-58.599, -23.0786) (-58.6254, -23.0962) (-58.6474, -23.1138) (-58.6649, -23.1314) knots 0 0 0 0 1 1 1 1
  spline S150 degree 3 poles (-58.1903, -22.7622) (-58.3134, -22.8501) (-58.4276, -22.938) (-58.5331, -23.0259) knots 0 0 0 0 1 1 1 1
  spline S151 degree 3 poles (-67.6033, -10.9367) (-67.6033, -10.9983) (-67.5945, -11.0466) (-67.5769, -11.0818) knots 0 0 0 0 1 1 1 1
  spline S152 degree 3 poles (-58.6649, -23.1314) (-58.8231, -23.2544) (-58.9769, -23.3862) (-59.1264, -23.5269) knots 0 0 0 0 1 1 1 1
  line L79 (-67.5769, -11.3454) -> (-67.5769, -11.4245)
  spline S153 degree 3 poles (-59.5614, -23.9487) (-59.9833, -24.3354) (-60.37, -24.7046) (-60.7215, -25.0561) knots 0 0 0 0 1 1 1 1
  spline S154 degree 3 poles (-57.8212, -22.4722) (-57.9442, -22.5777) (-58.0673, -22.6743) (-58.1903, -22.7622) knots 0 0 0 0 1 1 1 1
  spline S155 degree 3 poles (-57.7026, -22.3799) (-57.7465, -22.4063) (-57.786, -22.437) (-57.8212, -22.4722) knots 0 0 0 0 1 1 1 1
  spline S156 degree 3 poles (-67.5901, -10.4226) (-67.5989, -10.5456) (-67.6033, -10.6599) (-67.6033, -10.7654) knots 0 0 0 0 1 1 1 1
  spline S157 degree 3 poles (-58.5331, -23.0259) (-58.5507, -23.0435) (-58.5727, -23.0611) (-58.599, -23.0786) knots 0 0 0 0 1 1 1 1
  spline S158 degree 3 poles (-57.5839, -22.2876) (-57.6191, -22.3228) (-57.6586, -22.3535) (-57.7026, -22.3799) knots 0 0 0 0 1 1 1 1
  spline S159 degree 3 poles (-55.7119, -20.0992) (-55.7119, -20.2398) (-55.725, -20.3848) (-55.7514, -20.5342) knots 0 0 0 0 1 1 1 1
  line L80 (-58.4804, -10.0798) -> (-58.4936, -10.0666)
  spline S160 degree 3 poles (-57.2016, -9.7371) (-57.2631, -9.7898) (-57.3202, -9.8513) (-57.373, -9.9216) knots 0 0 0 0 1 1 1 1
  spline S161 degree 3 poles (-57.0038, -9.5789) (-57.0741, -9.6316) (-57.1401, -9.6843) (-57.2016, -9.7371) knots 0 0 0 0 1 1 1 1
  spline S162 degree 3 poles (-67.5242, -10.0535) (-67.5593, -10.1765) (-67.5813, -10.2995) (-67.5901, -10.4226) knots 0 0 0 0 1 1 1 1
  spline S163 degree 3 poles (-58.6254, -11.0027) (-58.6518, -10.9851) (-58.6737, -10.9499) (-58.6913, -10.8972) knots 0 0 0 0 1 1 1 1
  spline S164 degree 3 poles (-58.6913, -10.8576) (-58.6913, -10.8489) (-58.7001, -10.8357) (-58.7177, -10.8181) knots 0 0 0 0 1 1 1 1
  line L81 (-58.6913, -10.8972) -> (-58.6913, -10.8576)
  spline S165 degree 3 poles (-57.373, -9.9216) (-57.6542, -10.1853) (-57.8959, -10.4314) (-58.0981, -10.6599) knots 0 0 0 0 1 1 1 1
  spline S166 degree 3 poles (-58.0981, -10.6599) (-58.3002, -10.8884) (-58.454, -11.0114) (-58.5595, -11.029) knots 0 0 0 0 1 1 1 1
  spline S167 degree 3 poles (-58.5595, -11.029) (-58.5771, -11.029) (-58.599, -11.0202) (-58.6254, -11.0027) knots 0 0 0 0 1 1 1 1
  arc A17 (-212.8884, -6.4676) -> (-213.2444, -6.6258) centre (-207.3135, -19.4907) ccw
  spline S168 degree 3 poles (-214.365, -7.2058) (-214.2244, -7.118) (-214.0881, -7.0389) (-213.9563, -6.9685) knots 0 0 0 0 1 1 1 1
  spline S169 degree 3 poles (-214.6682, -7.3772) (-214.5715, -7.3157) (-214.4704, -7.2586) (-214.365, -7.2058) knots 0 0 0 0 1 1 1 1
  spline S170 degree 3 poles (-214.945, -7.5486) (-214.8572, -7.4959) (-214.7649, -7.4388) (-214.6682, -7.3772) knots 0 0 0 0 1 1 1 1
  arc A18 (-215.6174, -8.0364) -> (-215.9733, -8.2869) centre (-198.739, -32.3997) ccw
  spline S171 degree 3 poles (-212.8884, -6.4676) (-212.8357, -6.45) (-212.7786, -6.428) (-212.7171, -6.4017) knots 0 0 0 0 1 1 1 1
  spline S172 degree 3 poles (-201.5244, -18.0162) (-201.3134, -18.2623) (-201.0937, -18.5128) (-200.8652, -18.7677) knots 0 0 0 0 1 1 1 1
  arc A19 (-213.2444, -6.6258) -> (-213.574, -6.784) centre (-208.3418, -17.2619) ccw
  spline S173 degree 3 poles (-213.9563, -6.9685) (-213.8245, -6.8982) (-213.697, -6.8367) (-213.574, -6.784) knots 0 0 0 0 1 1 1 1
  line L82 (-212.0974, -26.0053) -> (-212.1502, -21.7603)
  spline S174 degree 3 poles (-215.2878, -7.7859) (-215.2351, -7.7508) (-215.178, -7.7156) (-215.1164, -7.6804) knots 0 0 0 0 1 1 1 1
  line L83 (-208.6434, -24.8188) -> (-212.0974, -26.0053)
  line L84 (-212.2293, -8.2605) -> (-215.9733, -8.2869)
  line L85 (-204.161, -5.8875) -> (-204.1479, -5.8875)
  spline S175 degree 3 poles (-215.1164, -7.6804) (-215.0549, -7.6453) (-214.9978, -7.6013) (-214.945, -7.5486) knots 0 0 0 0 1 1 1 1
  spline S176 degree 3 poles (-208.4325, -6.2435) (-207.9754, -6.1995) (-207.5272, -6.1512) (-207.0878, -6.0984) knots 0 0 0 0 1 1 1 1
  spline S177 degree 3 poles (-11.3683, -16.3024) (-11.3683, -15.1422) (-11.6672, -14.0568) (-12.2648, -13.0461) knots 0 0 0 0 1 1 1 1
  spline S178 degree 3 poles (-13.9523, -23.395) (-13.6359, -22.938) (-13.3546, -22.481) (-13.1085, -22.024) knots 0 0 0 0 1 1 1 1
  spline S179 degree 3 poles (-209.9617, -6.3357) (-209.3992, -6.3182) (-208.8895, -6.2874) (-208.4325, -6.2435) knots 0 0 0 0 1 1 1 1
  line L86 (-204.2006, -5.8875) -> (-204.161, -5.8875)
  spline S180 degree 3 poles (-210.6604, -6.3621) (-210.4407, -6.3621) (-210.2078, -6.3533) (-209.9617, -6.3357) knots 0 0 0 0 1 1 1 1
  line L87 (-19.3179, -7.9441) -> (-19.4893, -7.9441)
  spline S181 degree 3 poles (-211.8865, -6.3357) (-211.8338, -6.3533) (-211.7766, -6.3621) (-211.7151, -6.3621) knots 0 0 0 0 1 1 1 1
  line L88 (-212.5457, -6.3357) -> (-212.2029, -6.3357)
  spline S182 degree 3 poles (-18.0655, -8.2078) (-18.2061, -8.155) (-18.3687, -8.1067) (-18.5533, -8.0628) knots 0 0 0 0 1 1 1 1
  spline S183 degree 3 poles (-17.4063, -8.4187) (-17.4415, -8.4187) (-17.5162, -8.3967) (-17.6304, -8.3528) knots 0 0 0 0 1 1 1 1
  line L89 (-11.3683, -16.3683) -> (-11.3683, -16.3024)
  line L90 (-23.4707, -12.1364) -> (-23.4707, -24.6079)
  line L91 (-208.6434, -11.3191) -> (-208.6434, -24.8188)
  line L92 (-212.2029, -6.3357) -> (-211.8865, -6.3357)
  arc A20 (-215.6174, -8.0364) -> (-215.2878, -7.7859) centre (-218.2577, -4.2202) ccw
  spline S184 degree 3 poles (-19.1202, -7.9705) (-19.1905, -7.9529) (-19.2564, -7.9441) (-19.3179, -7.9441) knots 0 0 0 0 1 1 1 1
  line L93 (-211.5437, -6.3621) -> (-211.4251, -6.3621)
  line L94 (-211.3064, -6.3621) -> (-210.6604, -6.3621)
  line L95 (-211.7151, -6.3621) -> (-211.5437, -6.3621)
  line L96 (-208.617, -8.3396) -> (-208.6434, -11.3191)
  spline S185 degree 3 poles (-18.5533, -8.0628) (-18.7378, -8.0188) (-18.9268, -7.9881) (-19.1202, -7.9705) knots 0 0 0 0 1 1 1 1
  line L97 (-212.1502, -21.7603) -> (-212.2293, -8.2605)
  spline S186 degree 3 poles (-205.7562, -5.9798) (-205.2904, -5.9358) (-204.7851, -5.9051) (-204.2401, -5.8875) knots 0 0 0 0 1 1 1 1
  spline S187 degree 3 poles (-12.2648, -13.0461) (-12.8625, -12.0354) (-13.5128, -11.1872) (-14.2159, -10.5017) knots 0 0 0 0 1 1 1 1
  spline S188 degree 3 poles (-13.1085, -22.024) (-12.5812, -21.1275) (-12.1681, -20.2178) (-11.8693, -19.295) knots 0 0 0 0 1 1 1 1
  line L98 (-211.4251, -6.3621) -> (-211.3064, -6.3621)
  spline S189 degree 3 poles (-212.7171, -6.4017) (-212.6555, -6.3753) (-212.5984, -6.3533) (-212.5457, -6.3357) knots 0 0 0 0 1 1 1 1
  line L99 (-11.3683, -16.4606) -> (-11.3683, -16.3683)
  spline S190 degree 3 poles (-23.4311, -11.7014) (-23.4575, -11.8508) (-23.4707, -11.9958) (-23.4707, -12.1364) knots 0 0 0 0 1 1 1 1
  line L100 (-204.2401, -5.8875) -> (-204.2006, -5.8875)
  line L101 (-15.7452, -9.3679) -> (-17.4063, -8.4187)
  spline S191 degree 3 poles (-15.0069, -9.8425) (-15.2706, -9.6492) (-15.5167, -9.491) (-15.7452, -9.3679) knots 0 0 0 0 1 1 1 1
  spline S192 degree 3 poles (-11.8693, -19.295) (-11.5705, -18.3722) (-11.4035, -17.4274) (-11.3683, -16.4606) knots 0 0 0 0 1 1 1 1
  line L102 (-23.4707, -24.6079) -> (-27.0038, -25.9262)
  spline S193 degree 3 poles (-207.0878, -6.0984) (-206.6659, -6.0633) (-206.222, -6.0237) (-205.7562, -5.9798) knots 0 0 0 0 1 1 1 1
  spline S194 degree 3 poles (-17.6304, -8.3528) (-17.7447, -8.3089) (-17.8897, -8.2605) (-18.0655, -8.2078) knots 0 0 0 0 1 1 1 1
  spline S195 degree 3 poles (-14.2159, -10.5017) (-14.4796, -10.2556) (-14.7433, -10.0359) (-15.0069, -9.8425) knots 0 0 0 0 1 1 1 1
  spline S196 degree 3 poles (-105.5981, -16.9352) (-106.6439, -17.0055) (-107.7909, -17.0494) (-109.0389, -17.067) knots 0 0 0 0 1 1 1 1
  spline S197 degree 3 poles (-102.3681, -16.4606) (-102.4033, -16.4606) (-102.4428, -16.465) (-102.4868, -16.4738) knots 0 0 0 0 1 1 1 1
  spline S198 degree 3 poles (-114.0618, -18.2271) (-113.7014, -18.649) (-113.2928, -19.0885) (-112.8357, -19.5455) knots 0 0 0 0 1 1 1 1
  spline S199 degree 3 poles (-102.6054, -16.5133) (-103.5546, -16.7242) (-104.5522, -16.8649) (-105.5981, -16.9352) knots 0 0 0 0 1 1 1 1
  spline S200 degree 3 poles (-102.4868, -16.4738) (-102.5307, -16.4825) (-102.5703, -16.4957) (-102.6054, -16.5133) knots 0 0 0 0 1 1 1 1
  line L103 (-109.0389, -17.067) -> (-114.8923, -17.1197)
  spline S201 degree 3 poles (-130.4363, -8.2341) (-130.6209, -8.2166) (-130.8099, -8.2078) (-131.0032, -8.2078) knots 0 0 0 0 1 1 1 1
  arc A21 (-130.4363, -8.2341) -> (-129.8694, -8.2869) centre (-117.861, 123.8769) ccw
  spline S202 degree 3 poles (-127.18, -9.2361) (-127.9886, -8.7439) (-128.8851, -8.4275) (-129.8694, -8.2869) knots 0 0 0 0 1 1 1 1
  line L104 (-125.9672, -11.4509) -> (-125.9672, -11.385)
  spline S203 degree 3 poles (-116.2898, -21.4175) (-117.2741, -20.6441) (-117.9948, -19.7872) (-118.4518, -18.8468) knots 0 0 0 0 1 1 1 1
  spline S204 degree 3 poles (-67.3528, -9.4338) (-67.4319, -9.636) (-67.489, -9.8425) (-67.5242, -10.0535) knots 0 0 0 0 1 1 1 1
  spline S205 degree 3 poles (-61.9344, -8.946) (-62.1454, -8.9109) (-62.3475, -8.8845) (-62.5409, -8.8669) knots 0 0 0 0 1 1 1 1
  arc A22 (-63.2791, -8.7878) -> (-64.0701, -8.7615) centre (-64.0705, -20.6496) ccw
  line L105 (-61.3016, -9.0515) -> (-61.9344, -8.946)
  spline S206 degree 3 poles (-100.7993, -22.9995) (-100.8257, -23.0171) (-100.8564, -23.0347) (-100.8916, -23.0523) knots 0 0 0 0 1 1 1 1
  spline S207 degree 3 poles (-100.3643, -22.1953) (-100.083, -22.0284) (-99.9424, -21.98) (-99.9424, -22.0503) knots 0 0 0 0 1 1 1 1
  spline S208 degree 3 poles (-106.4154, -23.4082) (-105.8617, -23.5576) (-105.2773, -23.6323) (-104.662, -23.6323) knots 0 0 0 0 1 1 1 1
  spline S209 degree 3 poles (-64.4656, -8.7615) (-64.9754, -8.7615) (-65.4456, -8.7747) (-65.8762, -8.801) knots 0 0 0 0 1 1 1 1
  spline S210 degree 3 poles (-62.5409, -8.8669) (-62.7694, -8.8318) (-63.0155, -8.8054) (-63.2791, -8.7878) knots 0 0 0 0 1 1 1 1
  spline S211 degree 3 poles (-103.08, -23.4741) (-102.9394, -23.439) (-102.7856, -23.395) (-102.6186, -23.3423) knots 0 0 0 0 1 1 1 1
  spline S212 degree 3 poles (-118.4518, -18.8468) (-118.9089, -17.9064) (-119.1374, -16.8209) (-119.1374, -15.5905) knots 0 0 0 0 1 1 1 1
  spline S213 degree 3 poles (-100.2324, -22.5513) (-100.3027, -22.6216) (-100.3818, -22.6919) (-100.4697, -22.7622) knots 0 0 0 0 1 1 1 1
  spline S214 degree 3 poles (-65.8762, -8.801) (-66.3069, -8.8274) (-66.6189, -8.8582) (-66.8123, -8.8933) knots 0 0 0 0 1 1 1 1
  spline S215 degree 3 poles (-66.9968, -8.946) (-67.155, -9.0691) (-67.2737, -9.2317) (-67.3528, -9.4338) knots 0 0 0 0 1 1 1 1
  line L106 (-64.0701, -8.7615) -> (-64.2679, -8.7615)
  line L107 (-66.8123, -8.8933) -> (-66.9309, -8.9329)
  spline S216 degree 3 poles (-100.7334, -22.9468) (-100.751, -22.9644) (-100.7729, -22.982) (-100.7993, -22.9995) knots 0 0 0 0 1 1 1 1
  spline S217 degree 3 poles (-100.0215, -22.2876) (-100.0742, -22.3755) (-100.1445, -22.4634) (-100.2324, -22.5513) knots 0 0 0 0 1 1 1 1
  arc A23 (-102.6186, -23.3423) -> (-102.1308, -23.1577) centre (-104.0146, -18.9161) ccw
  spline S218 degree 3 poles (-101.7485, -22.96) (-101.6167, -22.8985) (-101.4892, -22.8325) (-101.3662, -22.7622) knots 0 0 0 0 1 1 1 1
  spline S219 degree 3 poles (-66.9309, -8.9329) (-66.9573, -8.9417) (-66.9793, -8.946) (-66.9968, -8.946) knots 0 0 0 0 1 1 1 1
  line L108 (-64.2679, -8.7615) -> (-64.4656, -8.7615)
  spline S220 degree 3 poles (-103.8974, -23.5928) (-103.6337, -23.5664) (-103.3613, -23.5269) (-103.08, -23.4741) knots 0 0 0 0 1 1 1 1
  spline S221 degree 3 poles (-101.3662, -22.7622) (-100.9795, -22.5513) (-100.6455, -22.3623) (-100.3643, -22.1953) knots 0 0 0 0 1 1 1 1
  spline S222 degree 3 poles (-100.4697, -22.7622) (-100.5576, -22.8325) (-100.6455, -22.8941) (-100.7334, -22.9468) knots 0 0 0 0 1 1 1 1
  spline S223 degree 3 poles (-99.9424, -22.0503) (-99.9424, -22.1206) (-99.9688, -22.1997) (-100.0215, -22.2876) knots 0 0 0 0 1 1 1 1
  spline S224 degree 3 poles (-102.1308, -23.1577) (-102.0078, -23.0874) (-101.8803, -23.0215) (-101.7485, -22.96) knots 0 0 0 0 1 1 1 1
  spline S225 degree 3 poles (-104.662, -23.6323) (-104.4159, -23.6323) (-104.1611, -23.6191) (-103.8974, -23.5928) knots 0 0 0 0 1 1 1 1
  spline S226 degree 3 poles (-108.0633, -22.7886) (-107.5184, -23.0523) (-106.9691, -23.2588) (-106.4154, -23.4082) knots 0 0 0 0 1 1 1 1
  arc A24 (-119.111, -14.7467) -> (-119.1374, -15.1686) centre (-115.7394, -15.1692) ccw
  line L109 (-119.1374, -15.5905) -> (-119.1374, -15.1686)
  line L110 (-113.2049, -23.9487) -> (-116.2898, -21.4175)
  spline S227 degree 3 poles (-83.4868, -8.2078) (-83.6274, -8.155) (-83.79, -8.1067) (-83.9745, -8.0628) knots 0 0 0 0 1 1 1 1
  spline S228 degree 3 poles (-101.0498, -15.4191) (-100.9092, -15.3927) (-100.7773, -15.3707) (-100.6543, -15.3532) knots 0 0 0 0 1 1 1 1
  line L111 (-103.3964, -15.6432) -> (-103.0932, -15.6432)
  spline S229 degree 3 poles (-55.6064, -7.6277) (-55.5185, -7.7683) (-55.5668, -7.9749) (-55.7514, -8.2473) knots 0 0 0 0 1 1 1 1
  line L112 (-81.4565, -26.1372) -> (-80.3755, -24.7397)
  line L113 (-82.0498, -26.8623) -> (-82.0102, -26.8227)
  spline S230 degree 3 poles (-112.0579, -24.7529) (-112.4534, -24.5156) (-112.8357, -24.2476) (-113.2049, -23.9487) knots 0 0 0 0 1 1 1 1
  spline S231 degree 3 poles (-106.2968, -25.8735) (-106.6483, -25.9262) (-107.0526, -25.9614) (-107.5096, -25.979) knots 0 0 0 0 1 1 1 1
  spline S232 degree 3 poles (-100.2456, -15.2477) (-100.1138, -15.2125) (-99.9688, -15.1686) (-99.8106, -15.1159) knots 0 0 0 0 1 1 1 1
  spline S233 degree 3 poles (-101.498, -15.5114) (-101.3398, -15.4762) (-101.1904, -15.4455) (-101.0498, -15.4191) knots 0 0 0 0 1 1 1 1
  spline S234 degree 3 poles (-55.7514, -8.2473) (-55.936, -8.5198) (-56.1865, -8.8142) (-56.5029, -9.1306) knots 0 0 0 0 1 1 1 1
  spline S235 degree 3 poles (-57.2543, -6.6653) (-56.5073, -6.8147) (-55.958, -7.1355) (-55.6064, -7.6277) knots 0 0 0 0 1 1 1 1
  spline S236 degree 3 poles (-88.7601, -11.24) (-88.7953, -11.3982) (-88.826, -11.552) (-88.8524, -11.7014) knots 0 0 0 0 1 1 1 1
  spline S237 degree 3 poles (-104.1347, -25.0561) (-104.3281, -25.1968) (-104.517, -25.311) (-104.7016, -25.3989) knots 0 0 0 0 1 1 1 1
  spline S238 degree 3 poles (-60.1678, -6.283) (-60.0975, -6.283) (-60.0228, -6.2874) (-59.9437, -6.2962) knots 0 0 0 0 1 1 1 1
  spline S239 degree 3 poles (-62.8836, -6.2171) (-62.6024, -6.2083) (-62.3123, -6.2039) (-62.0135, -6.2039) knots 0 0 0 0 1 1 1 1
  line L114 (-107.5096, -25.979) -> (-107.6678, -25.979)
  spline S240 degree 3 poles (-77.2906, -19.295) (-76.9917, -18.3722) (-76.8248, -17.4274) (-76.7896, -16.4606) knots 0 0 0 0 1 1 1 1
  spline S241 degree 3 poles (-110.8582, -25.3462) (-111.2625, -25.188) (-111.6624, -24.9902) (-112.0579, -24.7529) knots 0 0 0 0 1 1 1 1
  spline S242 degree 3 poles (-78.5298, -22.024) (-78.0025, -21.1275) (-77.5894, -20.2178) (-77.2906, -19.295) knots 0 0 0 0 1 1 1 1
  line L115 (-62.0135, -6.2039) -> (-61.8158, -6.2039)
  spline S243 degree 3 poles (-79.3735, -23.395) (-79.0571, -22.938) (-78.7759, -22.481) (-78.5298, -22.024) knots 0 0 0 0 1 1 1 1
  line L116 (-59.6801, -6.3357) -> (-59.6405, -6.3357)
  spline S244 degree 3 poles (-102.79, -15.6432) (-102.5966, -15.6432) (-102.3945, -15.63) (-102.1836, -15.6037) knots 0 0 0 0 1 1 1 1
  arc A25 (-60.1678, -6.283) -> (-60.8797, -6.2303) centre (-70.1839, -136.6682) ccw
  line L117 (-103.0932, -15.6432) -> (-102.79, -15.6432)
  spline S245 degree 3 poles (-107.826, -25.979) (-108.2831, -25.979) (-108.7709, -25.9306) (-109.2894, -25.834) knots 0 0 0 0 1 1 1 1
  spline S246 degree 3 poles (-105.2421, -25.6098) (-105.5937, -25.7329) (-105.9452, -25.8208) (-106.2968, -25.8735) knots 0 0 0 0 1 1 1 1
  spline S247 degree 3 poles (-56.5029, -9.1306) (-56.5732, -9.2009) (-56.6523, -9.2756) (-56.7402, -9.3547) knots 0 0 0 0 1 1 1 1
  line L118 (-115.6306, -13.9294) -> (-115.6833, -15.2213)
  spline S248 degree 3 poles (-61.6444, -6.2039) (-61.3807, -6.2039) (-61.1258, -6.2127) (-60.8797, -6.2303) knots 0 0 0 0 1 1 1 1
  spline S249 degree 3 poles (-63.6219, -6.2303) (-63.411, -6.2303) (-63.1649, -6.2259) (-62.8836, -6.2171) knots 0 0 0 0 1 1 1 1
  line L119 (-100.8916, -23.0523) -> (-104.1347, -25.0561)
  arc A26 (-81.4565, -26.1372) -> (-81.7202, -26.4668) centre (-73.1448, -33.0568) ccw
  spline S250 degree 3 poles (-82.0102, -26.8227) (-81.9048, -26.6997) (-81.8081, -26.581) (-81.7202, -26.4668) knots 0 0 0 0 1 1 1 1
  spline S251 degree 3 poles (-80.3755, -24.7397) (-80.0239, -24.3003) (-79.6899, -23.8521) (-79.3735, -23.395) knots 0 0 0 0 1 1 1 1
  spline S252 degree 3 poles (-104.7016, -25.3989) (-104.8862, -25.4868) (-105.0663, -25.5571) (-105.2421, -25.6098) knots 0 0 0 0 1 1 1 1
  spline S253 degree 3 poles (-82.063, -26.9018) (-82.063, -26.8842) (-82.0586, -26.871) (-82.0498, -26.8623) knots 0 0 0 0 1 1 1 1
  line L120 (-81.5884, -27.4555) -> (-81.6938, -27.561)
  spline S254 degree 3 poles (-83.144, -28.4574) (-83.1791, -28.352) (-83.0781, -28.1498) (-82.8408, -27.851) knots 0 0 0 0 1 1 1 1
  spline S255 degree 3 poles (-82.6826, -28.3915) (-82.955, -28.5761) (-83.1088, -28.5981) (-83.144, -28.4574) knots 0 0 0 0 1 1 1 1
  spline S256 degree 3 poles (-81.7993, -27.6664) (-82.1157, -27.9653) (-82.4101, -28.207) (-82.6826, -28.3915) knots 0 0 0 0 1 1 1 1
  arc A27 (-100.6543, -15.3532) -> (-100.2456, -15.2477) centre (-107.2048, 10.8745) ccw
  line L121 (-61.8158, -6.2039) -> (-61.6444, -6.2039)
  line L122 (-81.6938, -27.561) -> (-81.7993, -27.6664)
  arc A28 (-85.1742, -7.9573) -> (-85.4379, -7.9968) centre (-84.9019, -10.6714) ccw
  spline S257 degree 3 poles (-59.9437, -6.2962) (-59.8646, -6.305) (-59.7899, -6.3182) (-59.7196, -6.3357) knots 0 0 0 0 1 1 1 1
  spline S258 degree 3 poles (-109.2894, -25.834) (-109.8079, -25.7373) (-110.3309, -25.5747) (-110.8582, -25.3462) knots 0 0 0 0 1 1 1 1
  line L123 (-107.6678, -25.979) -> (-107.826, -25.979)
  arc A29 (-84.9106, -7.9441) -> (-85.1742, -7.9573) centre (-84.9103, -10.5923) ccw
  line L124 (-103.7919, -15.6432) -> (-103.3964, -15.6432)
  spline S259 degree 3 poles (-59.6405, -6.3357) (-58.7968, -6.4061) (-58.0014, -6.5159) (-57.2543, -6.6653) knots 0 0 0 0 1 1 1 1
  spline S260 degree 3 poles (-87.4681, -9.1834) (-88.1009, -9.8162) (-88.5316, -10.5017) (-88.7601, -11.24) knots 0 0 0 0 1 1 1 1
  spline S261 degree 3 poles (-81.061, -26.9809) (-81.2192, -27.1391) (-81.395, -27.2973) (-81.5884, -27.4555) knots 0 0 0 0 1 1 1 1
  spline S262 degree 3 poles (-82.8408, -27.851) (-82.6035, -27.5522) (-82.3442, -27.2358) (-82.063, -26.9018) knots 0 0 0 0 1 1 1 1
  arc A30 (-104.2138, -15.6168) -> (-103.7919, -15.6432) centre (-103.7913, -12.2452) ccw
  line L125 (-84.7392, -7.9441) -> (-84.9106, -7.9441)
  spline S263 degree 3 poles (-84.5414, -7.9705) (-84.6117, -7.9529) (-84.6777, -7.9441) (-84.7392, -7.9441) knots 0 0 0 0 1 1 1 1
  line L126 (-115.6833, -15.2213) -> (-104.2138, -15.6168)
  line L127 (-59.7196, -6.3357) -> (-59.6801, -6.3357)
  spline S264 degree 3 poles (-102.1836, -15.6037) (-101.9726, -15.5773) (-101.7441, -15.5465) (-101.498, -15.5114) knots 0 0 0 0 1 1 1 1
  spline S265 degree 3 poles (-56.7402, -9.3547) (-56.8281, -9.4338) (-56.9159, -9.5085) (-57.0038, -9.5789) knots 0 0 0 0 1 1 1 1
  spline S266 degree 3 poles (-85.4379, -7.9968) (-86.1586, -8.155) (-86.8353, -8.5505) (-87.4681, -9.1834) knots 0 0 0 0 1 1 1 1
  spline S267 degree 3 poles (-83.9745, -8.0628) (-84.1591, -8.0188) (-84.3481, -7.9881) (-84.5414, -7.9705) knots 0 0 0 0 1 1 1 1
  spline S268 degree 3 poles (-117.5554, -9.6052) (-117.5378, -9.5876) (-117.5202, -9.5745) (-117.5026, -9.5657) knots 0 0 0 0 1 1 1 1
  spline S269 degree 3 poles (-87.9691, -8.7087) (-87.723, -8.5681) (-87.4681, -8.4187) (-87.2045, -8.2605) knots 0 0 0 0 1 1 1 1
  spline S270 degree 3 poles (-81.8125, -5.993) (-81.7861, -5.993) (-81.7641, -5.9842) (-81.7466, -5.9666) knots 0 0 0 0 1 1 1 1
  spline S271 degree 3 poles (-76.3677, -22.3535) (-76.7193, -22.7315) (-77.0005, -23.0259) (-77.2115, -23.2368) knots 0 0 0 0 1 1 1 1
  spline S272 degree 3 poles (-83.9218, -6.6126) (-83.122, -6.2874) (-82.4409, -6.0809) (-81.8784, -5.993) knots 0 0 0 0 1 1 1 1
  spline S273 degree 3 poles (-118.9265, -13.4284) (-118.7858, -12.6022) (-118.5881, -11.8288) (-118.3332, -11.1081) knots 0 0 0 0 1 1 1 1
  spline S274 degree 3 poles (-74.4957, -10.9763) (-73.4762, -12.3649) (-72.9664, -13.8327) (-72.9664, -15.3795) knots 0 0 0 0 1 1 1 1
  spline S275 degree 3 poles (-79.6372, -10.5017) (-79.9009, -10.2556) (-80.1645, -10.0359) (-80.4282, -9.8425) knots 0 0 0 0 1 1 1 1
  line L128 (-81.8784, -5.993) -> (-81.8125, -5.993)
  line L129 (-97.092, -8.3132) -> (-93.7962, -6.573)
  spline S276 degree 3 poles (-100.4697, -7.5222) (-100.0127, -7.6453) (-99.5908, -7.8035) (-99.2041, -7.9968) knots 0 0 0 0 1 1 1 1
  line L130 (-117.4499, -9.5261) -> (-117.4499, -9.4998)
  spline S277 degree 3 poles (-102.8164, -9.4998) (-103.2734, -9.3767) (-103.7568, -9.2976) (-104.2665, -9.2625) knots 0 0 0 0 1 1 1 1
  line L131 (-76.7896, -16.4606) -> (-76.7896, -16.3683)
  spline S278 degree 3 poles (-102.3418, -7.1531) (-102.2715, -7.1707) (-102.0517, -7.2058) (-101.6826, -7.2586) knots 0 0 0 0 1 1 1 1
  spline S279 degree 3 poles (-75.2603, -21.022) (-75.647, -21.5318) (-76.0162, -21.9756) (-76.3677, -22.3535) knots 0 0 0 0 1 1 1 1
  spline S280 degree 3 poles (-101.7353, -10.3699) (-101.999, -9.9128) (-102.3593, -9.6228) (-102.8164, -9.4998) knots 0 0 0 0 1 1 1 1
  line L132 (-104.7939, -9.2097) -> (-110.2518, -8.5769)
  spline S281 degree 3 poles (-98.5977, -8.7615) (-98.5977, -8.8845) (-98.6284, -9.0076) (-98.69, -9.1306) knots 0 0 0 0 1 1 1 1
  arc A31 (-111.1746, -8.511) -> (-112.0711, -8.4714) centre (-112.0717, -18.666) ccw
  spline S282 degree 3 poles (-101.3398, -11.7146) (-101.3398, -11.486) (-101.3706, -11.2619) (-101.4321, -11.0422) knots 0 0 0 0 1 1 1 1
  spline S283 degree 3 poles (-80.4282, -9.8425) (-80.6919, -9.6492) (-80.938, -9.491) (-81.1665, -9.3679) knots 0 0 0 0 1 1 1 1
  line L133 (-93.7962, -6.573) -> (-88.7601, -6.573)
  spline S284 degree 3 poles (-99.2041, -7.9968) (-98.8174, -8.1902) (-98.6153, -8.4363) (-98.5977, -8.7351) knots 0 0 0 0 1 1 1 1
  spline S285 degree 3 poles (-101.6826, -7.2586) (-101.3135, -7.3113) (-100.9092, -7.3992) (-100.4697, -7.5222) knots 0 0 0 0 1 1 1 1
  spline S286 degree 3 poles (-113.0203, -8.5374) (-113.3191, -8.5813) (-113.6179, -8.6648) (-113.9168, -8.7878) knots 0 0 0 0 1 1 1 1
  spline S287 degree 3 poles (-77.6861, -13.0461) (-78.2837, -12.0354) (-78.9341, -11.1872) (-79.6372, -10.5017) knots 0 0 0 0 1 1 1 1
  spline S288 degree 3 poles (-87.2045, -8.2605) (-86.9408, -8.1023) (-86.6771, -7.9529) (-86.4135, -7.8123) knots 0 0 0 0 1 1 1 1